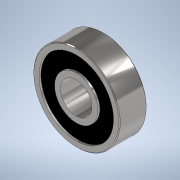
# Autodesk Inventor part: 608 Bearing
Saved by Autodesk Inventor 2022 (Build 260153000, 153)
## iProperties
Created: 2022-08-13
Part Number: 608 Bearing
Material: Generic
Document SubType Name: Modeling
Designer: Nick
Density: 1 g/cm^3
Appearance: Steel - Polished
Author: Nick
Autodesk Inventor part; units mm, degrees
ref_plane "YZ Plane" through (0, 0, 0) normal (1, 0, 0) x (0, 1, 0)
ref_plane "XZ Plane" through (0, 0, 0) normal (0, 1, 0) x (-1, 0, 0)
sketch "Sketch1" plane through (0, 0, 0) normal (0, 0, 1) x (1, 0, 0)
  circle A0 centre (0, 0) radius 4
  circle A1 centre (0, 0) radius 11
  dimension "d0" = 8
  dimension "d1" = 22
  constraints: 2 centre point, 2 coincident
  measures "d0" diameter of A0
  measures "d1" diameter of A1
extrude "Extrusion1" add sketch "Sketch1" along normal blind 7
sketch "Sketch2" plane through (0, 0, 7) normal (0, 0, 1) x (1, 0, 0)
  circle A0 centre (0, 0) radius 11 projected
  circle A1 centre (0, 0) radius 4 projected
  circle A2 centre (0, 0) radius 9.5
  circle A3 centre (0, 0) radius 5.5
  dimension "d4" = 1.5
  dimension "d5" = 1.5
  constraints: 2 centre point
  measures "d4" radial gap between concentric circles of A1 A3
  measures "d5" radial gap between concentric circles of A0 A2
extrude "Extrusion2" cut sketch "Sketch2" against normal blind 0.5 contours A2
ref_plane "Work Plane1" through (0, 0, 3.5) normal (0, 0, 1) x (1, 0, 0)
mirror "Mirror1" about plane through (0, 0, 3.5) normal (0, 0, 1) of "Extrusion2"
chamfer "Chamfer1" distance 0.2 angle 45 2 edges at (-11, 0, 7) (-11, 0, 0)
body "Solid1"
